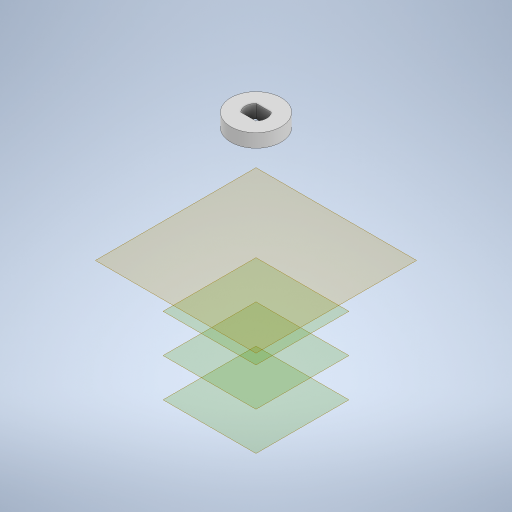
# Autodesk Inventor part: motor fit test
Saved by Autodesk Inventor 2024 (Build 280153020, 153B)
## iProperties
Created: 2024-02-08
Part Number: motor fit test
Material: Generic
Document SubType Name: Modeling
Designer: scottst
Density: 1 g/cm^3
Appearance: Default
Author: scottst
Autodesk Inventor part; units mm, degrees
ref_plane "YZ Plane" through (0, 0, 0) normal (1, 0, 0) x (0, 1, 0)
ref_plane "XZ Plane" through (0, 0, 0) normal (0, 1, 0) x (-1, 0, 0)
ref_plane "XY Plane" through (0, 0, 0) normal (0, 0, 1) x (1, 0, 0)
sketch "Sketch1" plane through (0, 0, 0) normal (0, 1, 0) x (-1, 0, 0)
  circle A0 centre (0, 0) radius 19.05
  dimension "d0" = 38.1
  constraints: 1 centre point, 1 coincident
  measures "d0" diameter of A0
extrude "Extrusion1" add sketch "Sketch1" along normal blind 67
sketch "Sketch2" plane through (0, 0, 0) normal (0, -1, 0) x (1, 0, 0)
  circle A0 centre (0, 0) radius 11.025
  dimension "d3" = 22.05
  constraints: 1 centre point, 1 coincident
  measures "d3" diameter of A0
extrude "Extrusion2" cut sketch "Sketch2" against normal blind 7
ref_plane "Work Plane1" through (0, 33.5, 0) normal (0, 1, 0) x (1, 0, 0)
ref_plane "Work Plane2" through (0, 22, 0) normal (0, -1, 0) x (1, 0, 0)
sketch "Sketch4" plane through (0, 22, 0) normal (0, -1, 0) x (1, 0, 0)
  circle A0 centre (0, 0) radius 13.97
  dimension "d7" = 27.94
  constraints: 1 centre point, 1 coincident
  measures "d7" diameter of A0
sketch "Sketch5" plane through (0, 7, 0) normal (0, -1, 0) x (1, 0, 0)
  circle A0 centre (0, 0) radius 11.025 projected
  circle A1 centre (0, 0) radius 11.025
  constraints: 1 centre point, 1 coincident
ref_plane "Work Plane3" through (0, 2, 0) normal (0, -1, 0) x (1, 0, 0)
ref_plane "Work Plane4" through (0, 12, 0) normal (0, -1, 0) x (1, 0, 0)
sketch "Sketch8" plane through (0, 12, 0) normal (0, -1, 0) x (1, 0, 0)
  circle A0 centre (0, 0) radius 9.5
  dimension "d11" = 19
  constraints: 1 centre point, 1 coincident
  measures "d11" diameter of A0
sketch "Sketch9" plane through (0, 33.5, 0) normal (0, 1, 0) x (1, 0, 0)
  circle A0 centre (0, 0) radius 13.97
  dimension "d12" = 27.94
  constraints: 1 centre point, 1 coincident
  measures "d12" diameter of A0
loft "Loft1" cut profiles "Sketch5", "Sketch8", "Sketch4", "Sketch9"
mirror "Mirror1" about plane through (0, 33.5, 0) normal (0, 1, 0) of "Loft1", "Extrusion2"
sketch "Sketch10" plane through (0, 67, 0) normal (0, 1, 0) x (1, 0, 0)
  circle A0 centre (0, 0) radius 16.3911
  constraints: 1 centre point, 1 coincident
extrude "Extrusion3" add sketch "Sketch10" against normal blind 12.7
sketch "Sketch12" plane through (0, 67, 0) normal (0, 1, 0) x (1, 0, 0)
  circle A0 centre (0, 0) radius 2.8
  line L0 (0, 0) -> (0, 2) construction
  line L1 (0, 0) -> (0, -2) construction
  line L2 (0, 2) -> (-1.9596, 2)
  line L3 (0, 2) -> (1.9596, 2)
  line L4 (0, -2) -> (-1.9596, -2)
  line L5 (0, -2) -> (1.9596, -2)
  dimension "d23" = 5.6
  dimension "d24" = 2
  dimension "d25" = 2
  constraints: 12 end point, 4 point on circle, 2 horizontal, 2 point on line, 2 vertical, 1 centre point, 1 coincident
  measures "d23" diameter of A0
  measures "d24" distance of L0.start L0.end
  measures "d25" distance of L0.start L1.end
extrude "Extrusion4" cut sketch "Sketch12" against normal blind 10 contours A0 L5 L4 L2 L3
sketch "Sketch13" plane through (0, 0, 0) normal (0, -1, 0) x (1, 0, 0)
  circle A0 centre (0, 0) radius 13.97 projected
  circle A1 centre (0, 0) radius 28.9364
  point P0 (13.97, 0)
  constraints: 1 centre point, 1 coincident, 1 horizontal alignment
extrude "Extrusion5" cut sketch "Sketch13" against normal blind 63.5 contours A0 | A1
sketch "Sketch14" plane through (0, 67, 0) normal (0, 1, 0) x (1, 0, 0)
  arc A0 (1.9596, -2) -> (1.9596, 2) centre (0, 0) ccw projected
  circle A1 centre (0, 0) radius 6.5686
  circle A2 centre (0, 0) radius 30.6019
  constraints: 2 centre point, 2 coincident
extrude "Extrusion6" cut sketch "Sketch14" against normal blind 63.5
body "Solid1"
